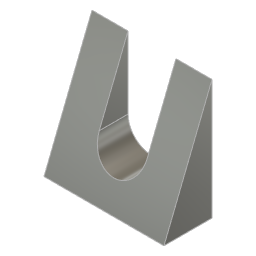
T5 Camera Wedge v2 (Autodesk Fusion 360 design; units mm, degrees)
Autodesk Fusion 360 part; units mm, degrees
sketch "Sketch1" plane through (0, 0, 0) normal (1, 0, 0) x (0, 0, -1)
  line L0 (9.4997, 47.4987) -> (9.4997, -2.5013)
  line L1 (9.4997, -2.5013) -> (-10.5003, -2.5013)
  line L2 (-10.5003, -2.5013) -> (9.4997, 47.4987)
  dimension "d1" = 50
  dimension "d2" = 20
  constraint vertical L0
  constraint perpendicular L0 L1
  measures "d1" distance of L0.start L0.end
  measures "d2" distance of L0.end L1.end
extrude "Extrude1" add sketch "Sketch1" along normal blind 50
sketch "Sketch2" plane through (0, 0, -9.4997) normal (0, 0, -1) x (-1, 0, 0)
  line L0 (0, -2.5013) -> (0, 47.4987)
  line L1 (0, 47.4987) -> (-50, 47.4987)
  line L2 (-50, 47.4987) -> (-50, -2.5013)
  line L3 (-50, -2.5013) -> (0, -2.5013)
  line L4 (-35, 47.4987) -> (-35, 17.4987)
  arc A0 (-35, 17.4987) -> (-15, 17.4987) centre (-25, 17.4987) ccw
  line L5 (-15, 17.4987) -> (-15, 47.4987)
  arc A1 (-15, 47.4987) -> (-35, 47.4987) centre (-25, 47.4987) ccw
  line L6 (-25, 47.4987) -> (-25, 17.4987) construction
  dimension "d5" = 20
  constraint tangent L4 A0
  constraint tangent A0 L5
  constraint parallel L4 L5
  constraint tangent L5 A1
  constraint tangent L4 A1
  constraint perpendicular L3 L6
  constraint midpoint L1 A1.centre
  measures "d5" diameter of A0
extrude "Extrude2" cut sketch "Sketch2" against normal through all contours L1 L4 A0 L5
